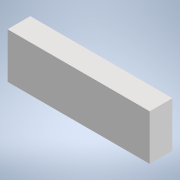
# Autodesk Inventor part: Battery
Saved by Autodesk Inventor 2020 (Build 240168000, 168)
## iProperties
Created: 2019-06-17
Part Number: Battery
Material: Acetal Resin, Black
Document SubType Name: Modeling
Designer: amirt
Density: 1.425 g/cm^3
Appearance: Smooth - Black
Author: amirt
Autodesk Inventor part; units mm, degrees
ref_plane "YZ Plane" through (0, 0, 0) normal (1, 0, 0) x (0, 1, 0)
ref_plane "XZ Plane" through (0, 0, 0) normal (0, 1, 0) x (-1, 0, 0)
ref_plane "XY Plane" through (0, 0, 0) normal (0, 0, 1) x (1, 0, 0)
sketch "Sketch1" plane through (0, 0, 0) normal (0, 0, 1) x (1, 0, 0)
  line L0 (-7.62, 20.32) -> (-1.27, 20.32) projected
  line L1 (2.54, 9.525) -> (2.54, -9.525) projected
  line L2 (-1.27, -20.32) -> (-7.62, -20.32) projected
  line L3 (2.54, 20.32) -> (-124.46, 20.32)
  line L4 (-124.46, 20.32) -> (-124.46, -20.32)
  line L5 (-124.46, -20.32) -> (2.54, -20.32)
  line L6 (2.54, -20.32) -> (2.54, 20.32)
  point P0 (0, 0)
  dimension "d0" = 127
  constraints: 8 end point, 2 parallel, 1 horizontal, 1 perpendicular
  measures "d0" distance of L5.end L4.end
extrude "Extrusion1" add sketch "Sketch1" along normal blind 20.32
body "Solid1"
